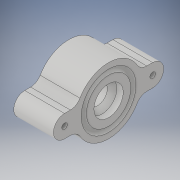
# Autodesk Inventor part: PeerIntput
Saved by Autodesk Inventor 2018 (Build 220112000, 112)
## iProperties
Created: 2020-03-28
Part Number: PeerIntput
Material: Generic
Document SubType Name: Modeling
Designer: emile
Density: 1 g/cm^3
Appearance: Default
Author: emile
Autodesk Inventor part; units mm, degrees
ref_plane "YZ Plane" through (0, 0, 0) normal (1, 0, 0) x (0, 1, 0)
ref_plane "XZ Plane" through (0, 0, 0) normal (0, 1, 0) x (-1, 0, 0)
ref_plane "XY Plane" through (0, 0, 0) normal (0, 0, 1) x (1, 0, 0)
sketch "Sketch2" plane through (0, 0, 0) normal (0, 0, 1) x (1, 0, 0)
  line L0 (-22.9183, 19.05) -> (22.9183, 19.05)
  line L1 (22.9183, 19.05) -> (22.9183, 0)
  line L2 (22.9183, 0) -> (-22.9183, 0)
  line L3 (-22.9183, 0) -> (-22.9183, 19.05)
  line L4 (-6.4083, 5.715) -> (-3.6778, 8.4455)
  line L5 (-6.4083, 5.715) -> (-22.9183, 5.715)
  line L6 (-3.6778, 8.4455) -> (0, 8.4455)
  line L7 (0, 8.4455) -> (0, 0)
  line L8 (0, 8.4455) -> (0, 19.05)
  circle A0 centre (0, 0) radius 7.9375 construction
  line L9 (-2.2089, 9.0164) -> (-4.3641, 6.8612) construction
  circle A1 centre (0, 14.2875) radius 1.524
  dimension "d10" = 19.05
  dimension "d11" = 16.51
  dimension "d35" = 45
  dimension "d36" = 0.635
  dimension "d37" = 15.875
  dimension "d38" = 5.715
  dimension "d39" = 8.4455
  dimension "d40" = 3.048
  dimension "d41" = 14.2875
  constraints: 20 end point, 3 parallel, 3 perpendicular, 2 centre point, 2 coincident, 2 horizontal, 2 midpoint, 2 point on line, 1 tangent
  measures "d10" distance between parallel lines of L2 L0
  measures "d11" distance from line of L3 L4.start
  measures "d35" angle of L6 L4
  measures "d36" distance between parallel lines of L4 L9
  measures "d37" diameter of A0
  measures "d38" distance between parallel lines of L2 L5
  measures "d39" distance between parallel lines of L2 L6
  measures "d40" diameter of A1
  measures "d41" distance from line of L2 A1.centre
revolve "Revolution1" add sketch "Sketch2" angle 360 about axis through (22.9183, 0, 0) along (-1, 0, 0) picked at (-0.475, 14.1074) contours L0 L8 A1 L6 L4 L5 L3 | L8 A1
sketch "Sketch3" plane through (0, 0, 0) normal (1, 0, 0) x (0, 0, -1)
  circle A0 centre (-25.4, 0) radius 1.5875
  line L0 (-25.4, -6.35) -> (-17.9605, -6.35)
  circle A1 centre (0, 0) radius 19.05 projected
  line L1 (-25.4, 6.35) -> (-17.9605, 6.35)
  arc A2 (-25.4, 6.35) -> (-25.4, -6.35) centre (-25.4, 0) ccw
  point P0 (0, 0)
  dimension "d20" = 3.175
  dimension "d21" = 25.4
  dimension "d22" = 12.7
  constraints: 4 end point, 4 point on circle, 2 centre point, 2 tangent, 1 coincident, 1 horizontal, 1 horizontal alignment, 1 parallel
  measures "d20" diameter of A0
  measures "d21" distance of point (0, 0) A0.centre
  measures "d22" distance between parallel lines of L0 L1
extrude "Extrusion2" add sketch "Sketch3" against normal up to surface (22.9183 mm away) contours A2 L1 A1 L0
fillet "Fillet1" radius 6.35 2 edges at (-11.4592, -6.35, 17.9605) (-11.4592, 6.35, 17.9605)
pattern_circular "Circular Pattern1" count 2 over 360 about axis through (-11.4592, 0, 0) along (1, 0, 0) of "Extrusion2", "Fillet1"
revolve "Revolution2" cut sketch "Sketch2" angle 360 about axis through (22.9183, 0, 0) along (-1, 0, 0) contours A1 L8 | L8 A1
body "Solid2"
